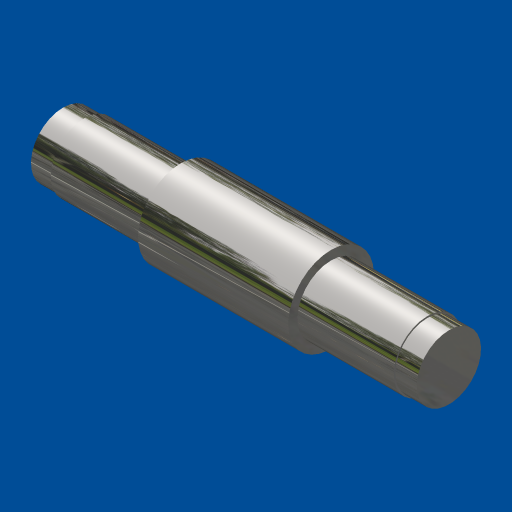
# Autodesk Inventor part: baseAxle
Saved by Autodesk Inventor 2023 (Build 270158030, 158C)
## iProperties
Created: 2023-03-03
Part Number: baseAxle
Material: Steel, Alloy
Document SubType Name: Modeling
Designer: kumpu
Density: 7.73 g/cm^3
Appearance: Semi-Polished
Author: kumpu
Autodesk Inventor part; units mm, degrees
ref_plane "YZ Plane" through (0, 0, 0) normal (1, 0, 0) x (0, 1, 0)
ref_plane "XZ Plane" through (0, 0, 0) normal (0, 1, 0) x (-1, 0, 0)
ref_plane "XY Plane" through (0, 0, 0) normal (0, 0, 1) x (1, 0, 0)
sketch "Sketch1" plane through (0, 0, 0) normal (0, 0, 1) x (1, 0, 0)
  line L0 (0, 12.7) -> (0, 0)
  line L1 (0, 0) -> (57.15, 0)
  line L2 (57.15, 0) -> (57.15, 9.525)
  line L3 (57.15, 9.525) -> (50.8, 9.525)
  line L4 (50.8, 9.525) -> (50.8, 10)
  line L5 (50.8, 10) -> (22.25, 10)
  line L6 (22.25, 10) -> (22.25, 12.7)
  line L7 (22.25, 12.7) -> (0, 12.7)
  dimension "d0" = 57.15
  dimension "d1" = 9.525
  dimension "d2" = 10
  dimension "d3" = 12.7
  dimension "d4" = 22.25
  dimension "d5" = 6.35
  constraints: 16 end point, 7 perpendicular, 1 coincident, 1 vertical
  measures "d0" distance of L0.end L1.end
  measures "d1" distance between parallel lines of L1 L3
  measures "d2" distance between parallel lines of L1 L5
  measures "d3" distance between parallel lines of L1 L7
  measures "d4" distance of L6.end L0.start
  measures "d5" distance of L2.end L3.end
revolve "Revolution1" add sketch "Sketch1" angle 360 about axis through (0, 0, 0) along (1, 0, 0)
mirror "Mirror1" about plane through (0, 0, 0) normal (1, 0, 0) of "Revolution1"
body "Solid1"
